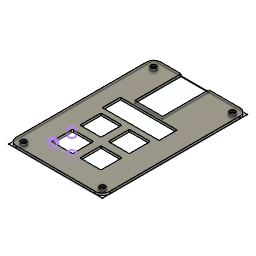
topplate v1 (Autodesk Fusion 360 design; units mm, degrees)
Autodesk Fusion 360 part; units mm, degrees
sketch "plate-2025-11-24T01_24_03.301Z" plane through (0, 0, 0) normal (0, 0, 1) x (1, 0, 0)
  line L0 (3.025, -2.525) -> (16.025, -2.525)
  line L1 (3.025, -16.525) -> (16.025, -16.525)
  line L2 (2.525, -3.025) -> (2.525, -16.025)
  line L3 (16.525, -3.025) -> (16.525, -16.025)
  arc A0 (3.025, -2.525) -> (2.525, -3.025) centre (3.025, -3.025) ccw
  arc A1 (16.525, -3.025) -> (16.025, -2.525) centre (16.025, -3.025) ccw
  arc A2 (2.525, -16.025) -> (3.025, -16.525) centre (3.025, -16.025) ccw
  arc A3 (16.025, -16.525) -> (16.525, -16.025) centre (16.025, -16.025) ccw
  line L4 (22.075, -2.525) -> (35.075, -2.525)
  line L5 (22.075, -16.525) -> (35.075, -16.525)
  line L6 (21.575, -3.025) -> (21.575, -16.025)
  line L7 (35.575, -3.025) -> (35.575, -16.025)
  arc A4 (22.075, -2.525) -> (21.575, -3.025) centre (22.075, -3.025) ccw
  arc A5 (35.575, -3.025) -> (35.075, -2.525) centre (35.075, -3.025) ccw
  arc A6 (21.575, -16.025) -> (22.075, -16.525) centre (22.075, -16.025) ccw
  arc A7 (35.075, -16.525) -> (35.575, -16.025) centre (35.075, -16.025) ccw
  line L8 (3.025, -21.575) -> (16.025, -21.575)
  line L9 (3.025, -35.575) -> (16.025, -35.575)
  line L10 (2.525, -22.075) -> (2.525, -35.075)
  line L11 (16.525, -22.075) -> (16.525, -35.075)
  arc A8 (3.025, -21.575) -> (2.525, -22.075) centre (3.025, -22.075) ccw
  arc A9 (16.525, -22.075) -> (16.025, -21.575) centre (16.025, -22.075) ccw
  arc A10 (2.525, -35.075) -> (3.025, -35.575) centre (3.025, -35.075) ccw
  arc A11 (16.025, -35.575) -> (16.525, -35.075) centre (16.025, -35.075) ccw
  line L12 (22.075, -21.575) -> (35.075, -21.575)
  line L13 (22.075, -35.575) -> (35.075, -35.575)
  line L14 (21.575, -22.075) -> (21.575, -35.075)
  line L15 (35.575, -22.075) -> (35.575, -35.075)
  arc A12 (22.075, -21.575) -> (21.575, -22.075) centre (22.075, -22.075) ccw
  arc A13 (35.575, -22.075) -> (35.075, -21.575) centre (35.075, -22.075) ccw
  arc A14 (21.575, -35.075) -> (22.075, -35.575) centre (22.075, -35.075) ccw
  arc A15 (35.075, -35.575) -> (35.575, -35.075) centre (35.075, -35.075) ccw
sketch "Sketch2" plane through (0, 0, 0) normal (0, 0, 1) x (1, 0, 0)
  line L0 (-11.896, 47.235) -> (50.966, 47.235)
  line L1 (50.966, 47.235) -> (50.966, -49.996)
  line L2 (50.966, -49.996) -> (-11.896, -49.996)
  line L3 (-11.896, -49.996) -> (-11.896, 47.235)
  line L4 (2.525, -22.075) -> (2.525, -35.075)
  line L5 (3.025, -35.575) -> (16.025, -35.575)
  circle A0 centre (-6.896, 42.235) radius 1.7
  circle A1 centre (45.966, 42.235) radius 1.7
  circle A2 centre (45.966, -44.996) radius 1.7
  circle A3 centre (-6.896, -44.996) radius 1.7
  line L6 (6.603, 47.235) -> (25.103, 47.235)
  line L7 (25.103, 47.235) -> (25.103, 16.235)
  line L8 (25.103, 16.235) -> (6.603, 16.235)
  line L9 (6.603, 16.235) -> (6.603, 47.235)
  dimension "d1" = 62.862
  dimension "d2" = 97.231
  dimension "d3" = 14.421
  dimension "d4" = 14.421
  dimension "d8" = 3.4
  dimension "d9" = 5
  dimension "d10" = 5
  dimension "d11" = 3.4
  dimension "d12" = 5
  dimension "d13" = 5
  dimension "d14" = 3.4
  dimension "d15" = 5
  dimension "d16" = 5
  dimension "d17" = 3.4
  dimension "d18" = 5
  dimension "d19" = 5
  dimension "d20" = 18.5
  dimension "d21" = 31
  dimension "d22" = 18.499
  constraint horizontal L0
  constraint vertical L1
  constraint horizontal L2
  constraint vertical L3
  constraint horizontal L6
  constraint vertical L7
  constraint horizontal L8
  constraint vertical L9
  constraint coincident L0 L6.start
  measures "d1" distance of L1 L3
  measures "d2" distance of L0 L2
  measures "d3" distance of L3 L4
  measures "d4" distance of L2 L5
  measures "d8" diameter of A0
  measures "d9" distance of L0 A0.centre
  measures "d10" distance of L3 A0.centre
  measures "d11" diameter of A1
  measures "d12" distance of L0 A1.centre
  measures "d13" distance of L1 A1.centre
  measures "d14" diameter of A2
  measures "d15" distance of L2 A2.centre
  measures "d16" distance of L1 A2.centre
  measures "d17" diameter of A3
  measures "d18" distance of L2 A3.centre
  measures "d19" distance of L3 A3.centre
  measures "d20" distance of L6.start L6.end
  measures "d21" distance of L6.start L8.end
  measures "d22" distance of L3 L9
extrude "Extrude1" add sketch "Sketch2" along normal blind 1.5 contours L0 L1 L2 L3 L7 L8 L9
extrude "Extrude2" cut sketch "plate-2025-11-24T01_24_03.301Z" along normal blind 1.5
fillet "Fillet1" radius 5 1 edges at (50.966, -49.996, 0.75)
fillet "Fillet2" radius 5 1 edges at (50.966, 47.235, 0.75)
fillet "Fillet3" radius 5 1 edges at (-11.896, 47.235, 0.75)
fillet "Fillet4" radius 5 1 edges at (-11.896, -49.996, 0.75)
sketch "Sketch3" plane through (0, 0, 1.5) normal (0, 0, 1) x (-1, 0, 0)
  arc A0 (11.896, 44.996) -> (6.896, 49.996) centre (6.896, 44.996) ccw
  line L0 (6.896, 49.996) -> (-45.966, 49.996)
  arc A1 (-45.966, 49.996) -> (-50.966, 44.996) centre (-45.966, 44.996) ccw
  line L1 (-50.966, 44.996) -> (-50.966, -42.235)
  arc A2 (-50.966, -42.235) -> (-45.966, -47.235) centre (-45.966, -42.235) ccw
  line L2 (-45.966, -47.235) -> (-25.103, -47.235)
  line L3 (-25.103, -47.235) -> (-25.103, -16.235)
  line L4 (-25.103, -16.235) -> (-6.603, -16.235)
  line L5 (-6.603, -16.235) -> (-6.603, -47.235)
  line L6 (-6.603, -47.235) -> (6.896, -47.235)
  arc A3 (6.896, -47.235) -> (11.896, -42.235) centre (6.896, -42.235) ccw
  line L7 (11.896, -42.235) -> (11.896, 44.996)
  line L8 (-22.075, 21.575) -> (-35.075, 21.575)
  arc A4 (-35.575, 22.075) -> (-35.075, 21.575) centre (-35.075, 22.075) ccw
  line L9 (-35.575, 22.075) -> (-35.575, 35.075)
  arc A5 (-35.075, 35.575) -> (-35.575, 35.075) centre (-35.075, 35.075) ccw
  line L10 (-35.075, 35.575) -> (-22.075, 35.575)
  arc A6 (-21.575, 35.075) -> (-22.075, 35.575) centre (-22.075, 35.075) ccw
  line L11 (-21.575, 35.075) -> (-21.575, 22.075)
  arc A7 (-22.075, 21.575) -> (-21.575, 22.075) centre (-22.075, 22.075) ccw
  line L12 (-3.025, 2.525) -> (-16.025, 2.525)
  arc A8 (-16.525, 3.025) -> (-16.025, 2.525) centre (-16.025, 3.025) ccw
  line L13 (-16.525, 3.025) -> (-16.525, 16.025)
  arc A9 (-16.025, 16.525) -> (-16.525, 16.025) centre (-16.025, 16.025) ccw
  line L14 (-16.025, 16.525) -> (-3.025, 16.525)
  arc A10 (-2.525, 16.025) -> (-3.025, 16.525) centre (-3.025, 16.025) ccw
  line L15 (-2.525, 16.025) -> (-2.525, 3.025)
  arc A11 (-3.025, 2.525) -> (-2.525, 3.025) centre (-3.025, 3.025) ccw
  line L16 (-3.025, 21.575) -> (-16.025, 21.575)
  arc A12 (-16.525, 22.075) -> (-16.025, 21.575) centre (-16.025, 22.075) ccw
  line L17 (-16.525, 22.075) -> (-16.525, 35.075)
  arc A13 (-16.025, 35.575) -> (-16.525, 35.075) centre (-16.025, 35.075) ccw
  line L18 (-16.025, 35.575) -> (-3.025, 35.575)
  arc A14 (-2.525, 35.075) -> (-3.025, 35.575) centre (-3.025, 35.075) ccw
  line L19 (-2.525, 35.075) -> (-2.525, 22.075)
  arc A15 (-3.025, 21.575) -> (-2.525, 22.075) centre (-3.025, 22.075) ccw
  line L20 (-22.075, 2.525) -> (-35.075, 2.525)
  arc A16 (-35.575, 3.025) -> (-35.075, 2.525) centre (-35.075, 3.025) ccw
  line L21 (-35.575, 3.025) -> (-35.575, 16.025)
  arc A17 (-35.075, 16.525) -> (-35.575, 16.025) centre (-35.075, 16.025) ccw
  line L22 (-35.075, 16.525) -> (-22.075, 16.525)
  arc A18 (-21.575, 16.025) -> (-22.075, 16.525) centre (-22.075, 16.025) ccw
  line L23 (-21.575, 16.025) -> (-21.575, 3.025)
  arc A19 (-22.075, 2.525) -> (-21.575, 3.025) centre (-22.075, 3.025) ccw
  circle A20 centre (6.896, -42.235) radius 1.7
  circle A21 centre (-45.966, 44.996) radius 1.7
  circle A22 centre (-45.966, -42.235) radius 1.7
  circle A23 centre (6.896, 44.996) radius 1.7
  line L24 (0.08, -13.128) -> (-37.92, -13.128)
  line L25 (-37.92, -13.128) -> (-37.92, -1.128)
  line L26 (-37.92, -1.128) -> (0.08, -1.128)
  line L27 (0.08, -1.128) -> (0.08, -13.128)
  line L28 (11.896, 49.996) -> (11.896, -47.235)
  dimension "d35" = 38
  dimension "d36" = 12
  dimension "d37" = 11.816
  constraint horizontal L24
  constraint vertical L25
  constraint horizontal L26
  constraint vertical L27
  measures "d35" distance of L24.start L24.end
  measures "d36" distance of L24.start L26.end
  measures "d37" distance of L27 L28
extrude "Extrude3" cut sketch "Sketch3" against normal blind 1.5 contours L24 L25 L26 L27
